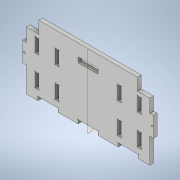
# Autodesk Inventor part: Side_one
Saved by Autodesk Inventor 2020 (Build 240168000, 168)
## iProperties
Created: 2019-12-17
Part Number: Side_one
Material: Generic
Document SubType Name: Modeling
Designer: fabfarm
Density: 1 g/cm^3
Appearance: Default
Author: fabfarm
Autodesk Inventor part; units mm, degrees
ref_plane "YZ Plane" through (0, 0, 0) normal (1, 0, 0) x (0, 1, 0)
ref_plane "XZ Plane" through (0, 0, 0) normal (0, 1, 0) x (-1, 0, 0)
ref_plane "XY Plane" through (0, 0, 0) normal (0, 0, 1) x (1, 0, 0)
sketch "Sketch1" plane through (0, 0, 0) normal (0, 0, 1) x (1, 0, 0)
  line L0 (0, 0) -> (-652, 0)
  line L1 (-652, 0) -> (-652, 350)
  line L2 (-652, 350) -> (0, 350)
  line L3 (0, 350) -> (0, 0)
  dimension "d0" = 350
  dimension "d1" = 652
  constraints: 8 end point, 2 parallel, 1 horizontal, 1 perpendicular
  measures "d0" distance of L2.end L0.start
  measures "d1" distance of L0.start L0.end
extrude "Extrusion1" add sketch "Sketch1" along normal blind 18.55
sketch "Sketch2" plane through (0, 0, 18.55) normal (0, 0, 1) x (1, 0, 0)
  line L0 (-652, 350) -> (-652, 0) projected
  line L1 (-652, 350) -> (-633.45, 350)
  line L2 (-633.45, 350) -> (-633.45, 224.9)
  line L3 (-633.45, 224.9) -> (-652, 224.9)
  line L4 (-652, 224.9) -> (-652, 350)
  line L5 (0, 350) -> (-652, 350) projected
  line L6 (-652, 0) -> (-633.45, 0)
  line L7 (-633.45, 0) -> (-633.45, 125.1)
  line L8 (-633.45, 125.1) -> (-652, 125.1)
  line L9 (-652, 125.1) -> (-652, 0)
  dimension "d54" = 18.55
  dimension "d55" = 125.1
  dimension "d57" = 125.1
  constraints: 16 end point, 4 parallel, 2 collinear, 2 horizontal, 2 perpendicular, 1 point on line
  measures "d54" distance of L1.start L1.end
  measures "d55" distance of L1.end L2.end
  measures "d57" distance of L6.end L7.end
extrude "Extrusion2" cut sketch "Sketch2" against normal blind 18.55
ref_plane "Work Plane1" through (-326, 0, 0) normal (1, 0, 0) x (0, 0, -1)
mirror "Mirror1" about plane through (-326, 0, 0) normal (1, 0, 0) of "Extrusion2"
sketch "Sketch3" plane through (0, 0, 18.55) normal (0, 0, 1) x (1, 0, 0)
  line L0 (0, 350) -> (-652, 350) projected
  line L1 (-652, 290) -> (-572, 290)
  line L2 (-572, 290) -> (-572, 350)
  line L3 (-572, 350) -> (-652, 350)
  line L4 (-652, 350) -> (-652, 290)
  line L5 (-652, 330) -> (-652, 350) construction
  line L6 (-652, 350) -> (-633.45, 350) construction
  point P0 (0, 0)
  point P1 (-18.55, 350)
  dimension "d19" = 80
  dimension "d22" = 60
  constraints: 12 end point, 3 perpendicular, 1 parallel, 1 point on line, 1 vertical
  measures "d19" distance of L0.end L2.end
  measures "d22" distance of L0.end L1.start
extrude "Extrusion3" cut sketch "Sketch3" against normal blind 18.55
mirror "Mirror2" about plane through (-326, 0, 0) normal (1, 0, 0) of "Extrusion3"
sketch "Sketch4" plane through (0, 0, 18.55) normal (0, 0, 1) x (1, 0, 0)
  line L0 (-633.45, 0) -> (-18.55, 0) projected
  line L1 (-576.1, 0) -> (-475.9, 0)
  line L2 (-475.9, 0) -> (-475.9, 18.55)
  line L3 (-475.9, 18.55) -> (-576.1, 18.55)
  line L4 (-576.1, 18.55) -> (-576.1, 0)
  line L5 (-376.1, 0) -> (-275.9, 0)
  line L6 (-275.9, 0) -> (-275.9, 18.55)
  line L7 (-275.9, 18.55) -> (-376.1, 18.55)
  line L8 (-376.1, 18.55) -> (-376.1, 0)
  line L9 (-633.45, 125.1) -> (-633.45, 0) projected
  line L10 (-176.1, 0) -> (-75.9, 0)
  line L11 (-75.9, 0) -> (-75.9, 18.55)
  line L12 (-75.9, 18.55) -> (-176.1, 18.55)
  line L13 (-176.1, 18.55) -> (-176.1, 0)
  line L14 (-18.55, 0) -> (-18.55, 125.1) projected
  line L15 (0, 125.1) -> (0, 224.9) projected
  line L16 (-652, 224.9) -> (-652, 125.1) projected
  point P0 (-75.9, 0)
  point P1 (-275.9, 0)
  point P2 (-475.9, 0)
  dimension "d59" = 100.2
  dimension "d60" = 100.2
  dimension "d61" = 99.8
  dimension "d62" = 99.8
  dimension "d63" = 100.2
  dimension "d66" = 18.55
  dimension "d67" = 75.9
  dimension "d68" = 75.9
  constraints: 24 end point, 6 parallel, 3 horizontal, 3 perpendicular, 3 point on line, 2 collinear
  measures "d59" distance of L2.end L3.end
  measures "d60" distance of L6.end L7.end
  measures "d61" distance between parallel lines of L2 L8
  measures "d62" distance between parallel lines of L13 L6
  measures "d63" distance of L11.end L12.end
  measures "d66" distance of L3.end L1.start
  measures "d67" distance between parallel lines of L15 L11
  measures "d68" distance between parallel lines of L4 L16
extrude "Extrusion4" cut sketch "Sketch4" against normal blind 20
sketch "Sketch5" plane through (0, 0, 18.55) normal (0, 0, 1) x (1, 0, 0)
  line L0 (-652, 30) -> (-633.45, 30)
  line L1 (-633.45, 30) -> (-633.45, 0)
  line L2 (-633.45, 0) -> (-652, 0)
  line L3 (-652, 0) -> (-652, 30)
  line L4 (-18.55, 30) -> (0, 30) projected
  line L5 (-18.55, 30) -> (0, 30)
  line L6 (0, 30) -> (0, 0)
  line L7 (0, 0) -> (-18.55, 0)
  line L8 (-18.55, 0) -> (-18.55, 30)
  line L9 (-633.45, 30) -> (-633.45, 10) projected
  line L10 (-652, 0) -> (-18.55, 0) projected
  point P0 (-611, 0)
  constraints: 16 end point, 4 parallel, 2 collinear, 2 horizontal, 2 perpendicular
extrude "Extrusion5" cut sketch "Sketch5" against normal blind 20
sketch "Sketch6" plane through (0, 0, 18.55) normal (0, 0, 1) x (1, 0, 0)
  line L0 (-276, 265) -> (-376, 265)
  line L1 (-376, 265) -> (-376, 290)
  line L2 (-376, 290) -> (-276, 290)
  line L3 (-276, 290) -> (-276, 265)
  line L4 (-276, 265) -> (-376, 290) construction
  line L5 (-376, 265) -> (-276, 290) construction
  line L6 (-326, 420) -> (-326, -70) projected
  line L7 (-80, 350) -> (-572, 350) projected
  point P0 (0, 0)
  point P1 (-326, 277.5)
  dimension "d38" = 25
  dimension "d39" = 100
  dimension "d40" = 60
  constraints: 12 end point, 2 midpoint, 2 parallel, 1 horizontal, 1 perpendicular, 1 point on line
  measures "d38" distance of L0.end L1.end
  measures "d39" distance of L1.end L2.end
  measures "d40" distance between parallel lines of L7 L2
extrude "Extrusion6" cut sketch "Sketch6" against normal blind 20
fillet "Fillet1" radius 4 4 edges at (-276, 290, 9.275) (-276, 265, 9.275) (-376, 290, 9.275) (-376, 265, 9.275)
sketch "Sketch7" plane through (0, 0, 18.55) normal (0, 0, 1) x (1, 0, 0)
  line L0 (-590.85, 48.65) -> (-572, 48.65)
  line L1 (-572, 48.65) -> (-572, 118.85)
  line L2 (-572, 118.85) -> (-590.85, 118.85)
  line L3 (-590.85, 118.85) -> (-590.85, 48.65)
  line L4 (-491, 48.65) -> (-472.15, 48.65)
  line L5 (-472.15, 48.65) -> (-472.15, 118.85)
  line L6 (-472.15, 118.85) -> (-491, 118.85)
  line L7 (-491, 118.85) -> (-491, 48.65)
  line L8 (-572, 350) -> (-572, 290) projected
  line L9 (-576.1, 18.55) -> (-475.9, 18.55) projected
  point P0 (0, 0)
  dimension "d44" = 81
  dimension "d45" = 18.85
  dimension "d46" = 70.2
  dimension "d72" = 30.1
  constraints: 16 end point, 4 parallel, 2 collinear, 2 horizontal, 2 perpendicular, 2 point on line
  measures "d44" distance between parallel lines of L7 L1
  measures "d45" distance of L1.end L2.end
  measures "d46" distance of L2.end L0.start
  measures "d72" distance between parallel lines of L9 L0
extrude "Extrusion7" cut sketch "Sketch7" against normal blind 20
mirror "Mirror3" about plane through (-326, 0, 0) normal (1, 0, 0) of "Extrusion7"
sketch "Esquisse8" plane through (0, 0, 0) normal (0, 0, -1) x (-1, 0, 0)
  line L0 (80, 199.8) -> (61.15, 199.8)
  line L1 (61.15, 199.8) -> (61.15, 270)
  line L2 (61.15, 270) -> (80, 270)
  line L3 (80, 270) -> (80, 199.8)
  line L4 (161, 270) -> (179.85, 270)
  line L5 (179.85, 270) -> (179.85, 199.8)
  line L6 (179.85, 199.8) -> (161, 199.8)
  line L7 (161, 199.8) -> (161, 270)
  line L8 (61.15, 48.65) -> (61.15, 118.85) projected
  line L9 (80, 118.85) -> (80, 48.65) projected
  line L10 (161, 48.65) -> (161, 118.85) projected
  line L11 (179.85, 118.85) -> (179.85, 48.65) projected
  line L12 (0, 270) -> (18.55, 270) projected
  point P0 (0, 0)
  dimension "d51" = 70.2
  constraints: 16 end point, 5 collinear, 4 parallel, 2 horizontal, 2 perpendicular, 2 point on line
  measures "d51" distance of L0.end L1.end
extrude "Extrusion8" cut sketch "Esquisse8" against normal blind 20
mirror "Symétrie4" about plane through (-326, 0, 0) normal (1, 0, 0) of "Extrusion8"
sketch "Esquisse9" plane through (0, 0, 18.55) normal (0, 0, 1) x (1, 0, 0)
  line L0 (-652, 224.9) -> (-633.45, 224.9) construction
  circle A0 centre (-633.45, 224.9) radius 1.585
  line L1 (-652, 125.1) -> (-633.45, 125.1) construction
  circle A1 centre (-633.45, 125.1) radius 1.585
  line L2 (-572, 199.8) -> (-572, 270) construction
  circle A2 centre (-572, 270) radius 1.585
  line L3 (-590.85, 270) -> (-572, 270) construction
  circle A3 centre (-590.85, 270) radius 1.585
  circle A4 centre (-590.85, 199.8) radius 1.585
  circle A5 centre (-572, 200) radius 1.585
  line L4 (-590.85, 118.85) -> (-572, 118.85) construction
  circle A6 centre (-590.85, 118.85) radius 1.585
  circle A7 centre (-572, 118.85) radius 1.585
  circle A8 centre (-590.85, 48.65) radius 1.585
  line L5 (-572, 48.65) -> (-590.85, 48.65) construction
  circle A9 centre (-572, 48.65) radius 1.585
  line L6 (-633.45, 290) -> (-572, 290) construction
  circle A10 centre (-572, 290) radius 1.585
  line L7 (-576.1, 18.55) -> (-475.9, 18.55) construction
  circle A11 centre (-576.1, 18.55) radius 1.585
  circle A12 centre (-475.9, 18.55) radius 1.585
  line L8 (-491, 48.65) -> (-472.15, 48.65) construction
  circle A13 centre (-491, 48.65) radius 1.585
  circle A14 centre (-472.15, 48.65) radius 1.585
  circle A15 centre (-491, 118.85) radius 1.585
  circle A16 centre (-472.15, 118.85) radius 1.585
  line L9 (-376.1, 18.55) -> (-275.9, 18.55) construction
  circle A17 centre (-376.1, 18.55) radius 1.585
  circle A18 centre (-491, 270) radius 1.585
  circle A19 centre (-472.15, 270) radius 1.585
  circle A20 centre (-491, 199.8) radius 1.585
  circle A21 centre (-472.15, 199.8) radius 1.585
  line L10 (-590.85, 48.65) -> (-590.85, 118.85) construction
  line L11 (-491, 270) -> (-472.15, 270) construction
  line L12 (-491, 199.8) -> (-491, 270) construction
  line L13 (-572, 350) -> (-80, 350) projected
  line L14 (-326, 350) -> (-326, 18.55) construction
  line L15 (0, 224.9) -> (-18.55, 224.9) construction
  circle A22 centre (-18.55, 224.9) radius 1.585
  line L16 (0, 125.1) -> (-18.55, 125.1) construction
  circle A23 centre (-18.55, 125.1) radius 1.585
  line L17 (-80, 199.8) -> (-80, 270) construction
  circle A24 centre (-80, 270) radius 1.585
  line L18 (-61.15, 270) -> (-80, 270) construction
  circle A25 centre (-61.15, 270) radius 1.585
  circle A26 centre (-61.15, 199.8) radius 1.585
  circle A27 centre (-80, 200) radius 1.585
  line L19 (-61.15, 118.85) -> (-80, 118.85) construction
  circle A28 centre (-61.15, 118.85) radius 1.585
  circle A29 centre (-80, 118.85) radius 1.585
  circle A30 centre (-61.15, 48.65) radius 1.585
  line L20 (-80, 48.65) -> (-61.15, 48.65) construction
  circle A31 centre (-80, 48.65) radius 1.585
  line L21 (-18.55, 290) -> (-80, 290) construction
  circle A32 centre (-80, 290) radius 1.585
  line L22 (-75.9, 18.55) -> (-176.1, 18.55) construction
  circle A33 centre (-75.9, 18.55) radius 1.585
  circle A34 centre (-176.1, 18.55) radius 1.585
  line L23 (-161, 48.65) -> (-179.85, 48.65) construction
  circle A35 centre (-161, 48.65) radius 1.585
  circle A36 centre (-179.85, 48.65) radius 1.585
  circle A37 centre (-161, 118.85) radius 1.585
  circle A38 centre (-179.85, 118.85) radius 1.585
  circle A39 centre (-275.9, 18.55) radius 1.585
  circle A40 centre (-161, 270) radius 1.585
  circle A41 centre (-179.85, 270) radius 1.585
  circle A42 centre (-161, 199.8) radius 1.585
  circle A43 centre (-179.85, 199.8) radius 1.585
  line L24 (-61.15, 48.65) -> (-61.15, 118.85) construction
  line L25 (-161, 270) -> (-179.85, 270) construction
  line L26 (-161, 199.8) -> (-161, 270) construction
  line L27 (-572, 118.85) -> (-572, 48.65) projected
  line L28 (-472.15, 270) -> (-472.15, 199.8) projected
  line L29 (-472.15, 199.8) -> (-491, 199.8) projected
  point P0 (0, 0)
  point P1 (-161, 48.65)
  point P2 (-179.85, 118.85)
  point P3 (-161, 118.85)
  dimension "d69" = 3.17
  constraints: 44 centre point, 32 symmetric about line, 26 end point, 21 equal radius, 12 point on line, 8 coincident, 2 midpoint, 22 other
  measures "d69" diameter of A7
extrude "Extrusion9" cut sketch "Esquisse9" against normal blind 20
sketch "Esquisse11" plane through (0, 0, 18.55) normal (0, 0, 1) x (1, 0, 0)
  line L0 (-635.035, 224.9) -> (-652, 224.9) projected
  line L1 (-643.5175, 224.9) -> (-643.5175, 125.1) construction
  line L2 (-635.035, 125.1) -> (-652, 125.1) projected
  circle A0 centre (-643.5175, 175) radius 4
  line L3 (0, 224.9) -> (-16.965, 224.9) projected
  line L4 (-8.4825, 224.9) -> (-8.4825, 125.1) construction
  line L5 (-16.965, 125.1) -> (0, 125.1) projected
  circle A1 centre (-8.4825, 175) radius 4
  point P0 (0, 0)
  dimension "d73" = 8
  constraints: 6 midpoint, 4 end point, 2 centre point, 1 equal radius
  measures "d73" diameter of A0
extrude "Extrusion10" cut sketch "Esquisse11" against normal blind 20
equation "\"d57\" = d55"
body "Solid1"
